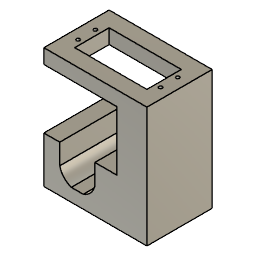
servo_mount (Autodesk Fusion 360 design; units mm, degrees)
Autodesk Fusion 360 part; units mm, degrees
note: some values were not read from the file. Set by a fixed rule: which sketch regions a step uses.
sketch "Sketch1" plane through (0, 0, 0) normal (0, 0, 1) x (1, 0, 0)
  line L0 (30, 19) -> (-30, 19)
  line L1 (-30, 19) -> (-30, -19)
  line L2 (-30, -19) -> (30, -19)
  line L3 (30, -19) -> (30, 19)
  line L4 (30, 19) -> (-30, -19) construction
  line L5 (-30, 19) -> (30, -19) construction
  line L6 (-21, -10) -> (21, -10)
  line L7 (21, -10) -> (21, 10)
  line L8 (21, 10) -> (-21, 10)
  line L9 (-21, 10) -> (-21, -10)
  line L10 (25, 9) -> (-25, 9) construction
  line L11 (-25, 9) -> (-25, -9) construction
  line L12 (-25, -9) -> (25, -9) construction
  line L13 (25, -9) -> (25, 9) construction
  line L14 (25, 9) -> (-25, -9) construction
  line L15 (-25, 9) -> (25, -9) construction
  line L16 (25, 9) -> (23, 9) construction
  line L17 (23, 9) -> (23, 5) construction
  line L18 (23, 5) -> (25, 5) construction
  line L19 (25, 5) -> (25, 9) construction
  circle A0 centre (24, 5) radius 1
  line L20 (25, -9) -> (23, -9) construction
  line L21 (23, -9) -> (23, -5) construction
  line L22 (23, -5) -> (25, -5) construction
  line L23 (25, -5) -> (25, -9) construction
  circle A1 centre (24, -5) radius 1
  line L24 (0, 19) -> (0, -19) construction
  circle A2 centre (-24, -5) radius 1
  circle A3 centre (-24, 5) radius 1
  dimension "d1" = 60
  dimension "d2" = 38
  dimension "d3" = -9
  dimension "d4" = 50
  dimension "d5" = 18
  dimension "d9" = 2
  dimension "d10" = 4
  dimension "d11" = 2
  dimension "d12" = 4
  constraint horizontal L0
  constraint perpendicular L0 L1
  constraint parallel L0 L2
  constraint parallel L1 L3
  constraint coincident L4 origin
  constraint coincident L5 origin
  constraint horizontal L10
  constraint perpendicular L10 L11
  constraint parallel L10 L12
  constraint parallel L11 L13
  constraint coincident L14 origin
  constraint coincident L15 origin
  constraint horizontal L16
  constraint vertical L17
  constraint horizontal L18
  constraint vertical L19
  constraint coincident L17.end A0
  constraint tangent L17 A0
  constraint coincident L18.end A0
  constraint horizontal L20
  constraint vertical L21
  constraint horizontal L22
  constraint vertical L23
  constraint coincident L21.end A1
  constraint tangent L21 A1
  constraint coincident L22.end A1
  constraint midpoint L0 L24.start
  constraint midpoint L2 L24.end
  constraint symmetric A0 L24 A3
  constraint symmetric A1 L24 A2
  measures "d1" distance of L1.end L2.end
  measures "d2" distance of L0.end L1.end
  measures "d4" distance of L11.end L12.end
  measures "d5" distance of L10.end L11.end
  measures "d9" distance of L10.start L16.end
  measures "d10" distance of L10.start L18.end
  measures "d11" distance of L12.end L20.end
  measures "d12" distance of L12.end L22.end
extrude "Extrude1" add sketch "Sketch1" along normal blind 8.5
sketch "Sketch2" plane through (0, 0, 0) normal (0, 0, 1) x (1, 0, 0)
  line L0 (30, -19) -> (30, 19)
  line L1 (-30, -19) -> (30, -19)
  line L2 (-30, 19) -> (-30, -19)
  line L3 (30, 19) -> (-30, 19)
  line L4 (30, 19) -> (12.5, 19)
  line L5 (12.5, 19) -> (12.5, -19)
  line L6 (12.5, -19) -> (30, -19)
  line L7 (30, -19) -> (30, 19)
  dimension "d15" = 17.5
  constraint horizontal L4
  constraint vertical L5
  constraint horizontal L6
  constraint vertical L7
  constraint coincident L1 L5.end
  constraint coincident L0.end L3.start
  measures "d15" distance of L0.end L4.end
extrude "Extrude2" add sketch "Sketch2" against normal blind 61.5 contours L0 L1 L3 L4 L5 L6 L7
sketch "Sketch3" plane through (0, 0, -61.5) normal (0, 0, -1) x (1, 0, 0)
  line L0 (30, -19) -> (30, 19)
  line L1 (30, 19) -> (12.5, 19)
  line L2 (12.5, 19) -> (12.5, -19) construction
  line L3 (12.5, -19) -> (30, -19)
  line L4 (-30, -19) -> (-30, 19)
  line L5 (30, -19) -> (-30, -19)
  line L6 (30, 19) -> (30, -19)
  line L7 (-30, 19) -> (30, 19)
  line L8 (0, -19) -> (0, 19)
  line L9 (-21, -19) -> (-21, 19)
  dimension "d18" = 30
  dimension "d19" = 9
  constraint coincident L5 L8.start
  constraint coincident L7 L8.end
  constraint perpendicular L7 L8
  constraint coincident L5 L9.start
  constraint coincident L7 L9.end
  constraint perpendicular L7 L9
  measures "d18" distance of L0 L8
  measures "d19" distance of L4 L9
extrude "Extrude3" add sketch "Sketch3" against normal blind 27
sketch "Sketch4" plane through (0, -19, 0) normal (0, -1, 0) x (1, 0, 0)
  line L0 (30, -61.5) -> (30, 8.5)
  line L1 (30, 8.5) -> (-30, 8.5)
  line L2 (-30, 8.5) -> (-30, 0)
  line L3 (-30, 0) -> (12.5, 0)
  line L4 (12.5, 0) -> (12.5, -34.5)
  line L5 (12.5, -34.5) -> (-30, -34.5)
  line L6 (-30, -34.5) -> (-30, -61.5)
  line L7 (-30, -61.5) -> (30, -61.5)
  line L8 (-21, -61.5) -> (0, -61.5) construction
  line L9 (0, -61.5) -> (0, -54.5) construction
  line L10 (0, -54.5) -> (-21, -54.5) construction
  line L11 (-21, -54.5) -> (-21, -61.5) construction
  line L12 (-10.5, -61.5) -> (-10.5, -54.5) construction
  line L13 (-21, -54.5) -> (-21, -44) construction
  line L14 (0, -44) -> (0, -54.5) construction
  line L15 (-21, -44) -> (0, -44) construction
  line L16 (-10.5, -54.5) -> (-10.5, -44) construction
  line L17 (-10.5, -53.8995) -> (-14, -53.8995)
  line L18 (-10.5, -53.8995) -> (-7, -53.8995)
  arc A0 (-21, -44) -> (-20.7222, -46.3995) centre (-10.5, -44) ccw construction
  arc A1 (-0.2778, -46.3995) -> (0, -44) centre (-10.5, -44) ccw construction
  arc A2 (-10.5, -54.5) -> (-7, -53.8995) centre (-10.5, -44) ccw construction
  arc A3 (-14, -53.8995) -> (-10.5, -54.5) centre (-10.5, -44) ccw construction
  line L19 (-21, -46.3995) -> (0, -46.3995) construction
  arc A4 (-20.7222, -46.3995) -> (-14, -53.8995) centre (-10.5, -44) ccw
  arc A5 (-7, -53.8995) -> (-0.2778, -46.3995) centre (-10.5, -44) ccw
  line L20 (-20.7222, -46.3995) -> (-20.7222, -33.3995)
  line L21 (-0.2778, -46.3995) -> (-0.2778, -33.3995)
  line L22 (-0.2778, -33.3995) -> (-20.7222, -33.3995)
  point P0 (0, -61.5)
  point P1 (-21, -61.5)
  dimension "d41" = 7
  dimension "d44" = 10.5
  dimension "d45" = 21
  dimension "d46" = 3.5
  dimension "d47" = 7.5
  dimension "d48" = 13
  dimension "d49" = 13
  constraint horizontal L8
  constraint vertical L9
  constraint horizontal L10
  constraint vertical L11
  constraint coincident P1 L8.start
  constraint coincident P0 L8.end
  constraint midpoint L8 L12.start
  constraint midpoint L10 L12.end
  constraint perpendicular L5 L13
  constraint coincident L16.end A0.centre
  constraint perpendicular L15 L16
  constraint coincident L16 L17.start
  constraint horizontal L17
  constraint coincident L18.end A0
  constraint perpendicular L16 L18
  constraint concentric A0 A1
  constraint concentric A0 A2
  constraint concentric A0 A3
  constraint coincident L13 L19.start
  constraint coincident L14 L19.end
  constraint perpendicular L14 L19
  constraint coincident L19 A0.end
  constraint concentric A0 A4
  constraint coincident L19 A1.start
  constraint concentric A1 A5
  constraint perpendicular L15 L20
  constraint perpendicular L15 L21
  measures "d41" distance of P1 L10.end
  measures "d44" distance of L10.end L13.end
  measures "d45" distance of L13.end L14.start
  measures "d46" distance of L17.start L17.end
  measures "d47" distance of L17 L19
  measures "d48" distance of A0.end L20.end
  measures "d49" distance of A1.start L21.end
extrude "Extrude4" cut sketch "Sketch4" against normal blind 38 contours L5 L17 L18 A4 A5 L20 L21
